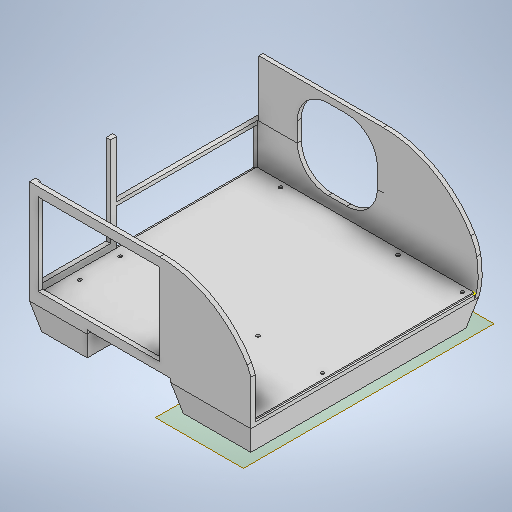
# Autodesk Inventor part: matx-arc-case-r2
Saved by Autodesk Inventor 2025 (Build 290162000, 162)
## iProperties
Created: 2024-07-20
Part Number: matx-arc-case-r2
Material: Generic
Document SubType Name: Modeling
Designer: admin
Density: 1 g/cm^3
Appearance: Default
Author: admin
Autodesk Inventor part; units mm, degrees
ref_plane "YZ Plane" through (0, 0, 0) normal (1, 0, 0) x (0, 1, 0)
ref_plane "XZ Plane" through (0, 0, 0) normal (0, 1, 0) x (-1, 0, 0)
ref_plane "XY Plane" through (0, 0, 0) normal (0, 0, 1) x (1, 0, 0)
sketch "Sketch2" plane through (0, 0, 0) normal (0, 1, 0) x (-1, 0, 0)
  line L0 (0, 0) -> (0, -243.84)
  line L1 (0, -243.84) -> (243.84, -243.84)
  line L2 (243.84, -243.84) -> (243.84, 0)
  line L3 (243.84, 0) -> (0, 0)
  line L4 (243.84, 0) -> (233.68, 0)
  line L5 (233.68, 0) -> (6.35, 0)
  line L6 (233.68, 0) -> (78.74, 0)
  line L7 (233.68, -243.84) -> (210.82, -243.84)
  line L8 (233.68, 0) -> (233.68, -243.84)
  line L9 (243.84, -243.84) -> (243.84, -85.09)
  line L10 (6.35, 0) -> (6.35, -243.84)
  line L11 (78.74, 0) -> (78.74, -243.84)
  line L12 (243.84, -85.09) -> (243.84, -31.85)
  line L13 (78.74, -31.85) -> (78.74, -77.57)
  line L14 (78.74, 0) -> (78.74, -34.29)
  line L15 (78.74, -34.29) -> (78.74, -13.97)
  line L16 (78.74, -34.29) -> (78.74, -80.01)
  circle A0 centre (78.74, -80.01) radius 2
  circle A1 centre (78.74, -34.29) radius 2
  circle A2 centre (78.74, -13.97) radius 2
  circle A3 centre (6.35, -80.01) radius 2
  line L17 (78.74, -34.29) -> (78.74, -237.49)
  circle A4 centre (78.74, -237.49) radius 2
  circle A5 centre (6.35, -237.49) radius 2
  circle A6 centre (210.82, -237.49) radius 2
  circle A7 centre (233.68, -34.29) radius 2
  circle A8 centre (233.68, -80.01) radius 2
  dimension "d79" = 243.84
  dimension "d80" = 243.84
  dimension "d81" = 10.16
  dimension "d82" = 227.33
  dimension "d83" = 154.94
  dimension "d84" = 22.86
  dimension "d85" = 158.75
  dimension "d92" = 34.29
  dimension "d93" = 20.32
  dimension "d94" = 45.72
  dimension "d95" = 203.2
  constraints: 36 end point, 17 point on line, 9 centre point, 4 coincident, 4 perpendicular, 2 vertical, 1 parallel
  measures "d79" distance of L0.start L0.end
  measures "d80" distance of L0.end L1.end
  measures "d81" distance of L2.end L4.end
  measures "d82" distance of L4.end L5.end
  measures "d83" distance of L4.end L6.end
  measures "d84" distance of L7.start L7.end
  measures "d85" distance of L1.end L9.end
  measures "d92" distance of L6.end L14.end
  measures "d93" distance of L14.end L15.end
  measures "d94" distance of L14.end L16.end
  measures "d95" distance of L17.start L17.end
extrude "Extrusion1" add sketch "Sketch2" along normal blind 1.5 contours L3 L10 A3 A5 L1 L0 | L3 L11 A2 A1 A0 A4 L1 L10 A5 A3 | L3 L8 A7 A8 L1 L11 A4 A0 A1 A2 | L3 L2 L1 L8 A8 A7
sketch "Sketch4" plane through (-243.84, 0, -243.84) normal (-1, 0, 0) x (0, 0, 1)
  line L0 (0.0105, -0.4083) -> (0.0105, -1.9083)
  line L1 (243.84, 0) -> (0, 0) projected
  line L2 (0.0105, -1.9083) -> (-1.25, -1.9083)
  line L3 (-1.25, -1.9083) -> (-1.25, 42.5417)
  line L4 (-1.25, -1.9083) -> (43.2, -1.9083) construction
  line L5 (-1.25, 42.5417) -> (157.5, 42.5417)
  line L6 (157.5, 42.5417) -> (157.5, -1.9083)
  line L7 (-1.25, -1.9083) -> (-1.25, -6.0083)
  line L8 (-1.25, -6.0083) -> (157.5, -6.0083)
  line L9 (-1.25, -6.0083) -> (-5.35, -6.0083)
  line L10 (-5.35, -6.0083) -> (-5.35, 42.5417)
  line L11 (-5.35, 42.5417) -> (-5.35, 46.6417)
  line L12 (-5.35, 46.6417) -> (157.5, 46.6417)
  line L13 (157.5, 46.6417) -> (161.6, 46.6417)
  line L14 (161.6, 46.6417) -> (161.6, -1.9083)
  line L15 (161.6, -6.0083) -> (157.5, -6.0083)
  line L16 (161.6, -6.0083) -> (161.6, -1.9083)
  line L17 (0.0105, -1.9083) -> (157.5, -1.9083)
  line L18 (161.6, -6.0083) -> (243.84, -6.0083)
  line L19 (161.6, -6.0083) -> (161.6, 9.1917)
  line L20 (161.6, 9.1917) -> (243.84, 9.1917)
  line L21 (243.84, 9.1917) -> (243.84, -6.0083)
  line L22 (157.5, 42.5417) -> (164.5, 42.5417)
  line L23 (164.5, 42.5417) -> (164.5, 9.1917)
  line L24 (164.5, 42.5417) -> (164.5, 46.6417)
  line L25 (164.5, 46.6417) -> (161.6, 46.6417)
  line L26 (164.5, 9.1917) -> (164.5, 110.1917)
  line L27 (164.5, 110.1917) -> (243.84, 110.1917)
  line L28 (243.84, 110.1917) -> (243.84, 9.1917)
  line L29 (157.5, 46.6417) -> (157.5, 110.1917)
  line L30 (250.84, 110.1917) -> (250.84, -6.0083)
  line L31 (250.84, -6.0083) -> (243.84, -6.0083)
  line L32 (243.84, 110.1917) -> (250.84, 110.1917)
  line L33 (157.5, 110.1917) -> (164.5, 110.1917)
  dimension "d98" = 1.5
  dimension "d103" = 44.45
  dimension "d104" = 90
  dimension "d105" = 158.75
  dimension "d106" = 4.1
  dimension "d107" = 4.1
  dimension "d108" = 4.1
  dimension "d109" = 4.1
  dimension "d110" = 15.2
  dimension "d111" = 7
  dimension "d112" = 101
  constraints: 66 end point, 14 perpendicular, 13 point on line, 3 horizontal, 3 vertical, 2 collinear, 2 parallel
  measures "d98" distance of L0.start L0.end
  measures "d103" distance of L2.end L3.end
  measures "d104" angle of L4 L3
  measures "d105" distance of L3.end L5.end
  measures "d106" distance of L2.end L7.end
  measures "d107" distance of L7.end L9.end
  measures "d108" distance of L10.end L11.end
  measures "d109" distance of L12.end L13.end
  measures "d110" distance of L15.start L19.end
  measures "d111" distance of L5.end L22.end
  measures "d112" distance of L23.end L26.end
extrude "Extrusion2" add sketch "Sketch4" along normal blind 5 contours L21 L18 L16 L14 L1 | L1 L14 L20 L21 | L21 L28 L32 L30 L31 | L14 L16 L15 L8 L7 L2 L17 L6 L1 | L1 L6 L22 L14 | L14 L22 L23 L20 | L5 L3 L7 L9 L10 L11 L12 L13 L14 L22 | L14 L25 L24 L22 | L26 L25 L13 L29 L33
sketch "Sketch5" plane through (-243.84, 0, -243.84) normal (1, 0, 0) x (0, 0, -1)
  line L0 (5.35, -6.0083) -> (-250.84, -6.0083) projected
  line L1 (-250.84, -6.0083) -> (5.35, -6.0083)
  line L2 (5.35, -6.0083) -> (5.35, -1.9083)
  line L3 (5.35, -1.9083) -> (-250.84, -1.9083)
  line L4 (-157.5, -1.9083) -> (1.25, -1.9083) projected
  line L5 (-250.84, -1.9083) -> (-250.84, -6.0083)
  point P0 (-243.84, 0)
  constraints: 8 end point, 2 collinear, 2 perpendicular
extrude "Extrusion3" add sketch "Sketch5" along normal blind 60
sketch "Sketch6" plane through (-248.84, -1.9083, -86.34) normal (0, 1, 0) x (1, 0, 0)
  circle A0 centre (15.16, -52.05) radius 2 projected
  circle A1 centre (15.16, -52.05) radius 2
  circle A2 centre (15.16, -6.33) radius 2 projected
  circle A3 centre (15.16, -6.33) radius 2
  circle A4 centre (37.9882, 151.128) radius 2.0223
  point P0 (248.84, -86.34)
  constraints: 3 centre point, 2 coincident
extrude "Extrusion4" cut sketch "Sketch6" against normal blind 28.25
ref_plane "Work Plane1" through (-248.84, -36.0083, -249.19) normal (0, -1, 0) x (1, 0, 0)
sketch "Sketch7" plane through (-248.84, -36.0083, -249.19) normal (0, -1, 0) x (1, 0, 0)
  line L0 (65, 256.19) -> (65, 0) projected
  line L1 (65, 256.19) -> (65, 249.19)
  line L2 (7, 249.19) -> (7, 7)
  line L3 (7, 7) -> (58, 7)
  line L4 (58, 7) -> (58, 249.19)
  line L5 (58, 249.19) -> (7, 249.19)
  line L6 (5, 249.19) -> (248.84, 249.19) projected
  dimension "d122" = 7
  constraints: 10 end point, 2 perpendicular, 1 collinear, 1 point on line
  measures "d122" distance of L1.end L4.end
loft "Loft1" add profiles "Sketch7" section 2 edges at (-216.34, -6.0083, 7) (-248.84, -6.0083, -121.095) (-216.34, -6.0083, -249.19) (-183.84, -6.0083, -121.095)
ref_plane "Work Plane2" through (0.16, 0, -243.84) normal (1, 0, 0) x (0, 0, -1)
sketch "Sketch8" plane through (0.16, 0, -243.84) normal (1, 0, 0) x (0, 0, -1)
  line L0 (5.35, -1.9083) -> (-250.84, -1.9083) projected
  line L1 (-250.84, -1.9083) -> (5.35, -1.9083)
  line L2 (5.35, -6.0083) -> (-250.84, -6.0083) projected
  line L3 (5.35, -1.9083) -> (5.35, -6.0083)
  line L4 (5.35, -6.0083) -> (-250.84, -6.0083)
  line L5 (-250.84, -6.0083) -> (-250.84, -1.9083)
  point P0 (-243.84, 0)
  constraints: 8 end point, 3 perpendicular, 1 horizontal
extrude "Extrusion5" add sketch "Sketch8" against normal blind 90
ref_plane "Work Plane3" through (0.16, -36.0083, -249.19) normal (0, -1, 0) x (1, 0, 0)
sketch "Sketch9" plane through (0.16, -36.0083, -249.19) normal (0, -1, 0) x (1, 0, 0)
  line L0 (0, 256.19) -> (-90, 256.19) projected
  line L1 (-90, 256.19) -> (-90, 0) projected
  line L2 (-83, 249.19) -> (-7, 249.19)
  line L3 (-7, 249.19) -> (-7, 7)
  line L4 (0, 0) -> (-90, 0) projected
  line L5 (-83, 7) -> (-7, 7)
  line L6 (-83, 7) -> (-83, 249.19)
  constraints: 8 end point, 1 perpendicular
loft "Loft2" add profiles "Sketch9" section 2 edges at (0.16, -6.0083, -121.095) (-44.84, -6.0083, 7) (-89.84, -6.0083, -121.095) (-44.84, -6.0083, -249.19)
sketch "Sketch10" plane through (-248.84, -1.9083, -86.34) normal (0, 1, 0) x (1, 0, 0)
  line L0 (5, 158.75) -> (5, 162.85) projected
  line L1 (242, 155.85) -> (249, 162.85) projected
  line L2 (5, 162.85) -> (249, 162.85)
  line L3 (249, 162.85) -> (249, 158.35)
  line L4 (249, 158.35) -> (5, 158.35)
  line L5 (5, 158.35) -> (5, 162.85)
  point P0 (248.84, -86.34)
  point P1 (244.5, 158.35)
  dimension "d142" = 4.5
  constraints: 8 end point, 3 perpendicular, 1 horizontal
  measures "d142" distance of L1.end L3.end
extrude "Extrusion6" add sketch "Sketch10" along normal blind 48.54
sketch "Sketch11" plane through (-183.84, -1.9083, -244.69) normal (0, 0, 1) x (1, 0, 0)
  point P0 (183.84, 1.9083)
sketch "Sketch12" plane through (-183.84, -6.0083, -249.19) normal (0, 0, -1) x (-1, 0, 0)
  line L0 (65, 116.2) -> (65, 52.65) projected
  line L1 (65, 52.65) -> (65, 116.2)
  line L2 (65, 116.2) -> (58.6377, 116.2)
  line L3 (58.6377, 116.2) -> (58.6377, 52.65)
  line L4 (58.6377, 52.65) -> (-81.3623, 52.64)
  line L5 (60, 52.64) -> (-184, 52.64) projected
  line L6 (58.6377, 116.2) -> (-81.3623, 116.2)
  line L7 (-81.3623, 116.2) -> (-81.3623, 52.64)
  line L8 (-179.5, 52.64) -> (-184, 52.64) projected
  arc A0 (-81.3623, 116.2) -> (-184, 52.64) centre (-81.3623, 1.5495) ccw
  line L9 (-184, 4.1) -> (-184, 52.64) projected
  arc A1 (-184, 52.64) -> (-184, -0.3678) centre (-99.2421, 26.1361) ccw
  line L10 (-184, -0.3678) -> (-184, 52.64)
  line L11 (-184, 4.1) -> (-184, 0) projected
  point P0 (-183.84, 6.0083)
  dimension "d145" = 140
  constraints: 14 end point, 4 point on circle, 3 perpendicular, 2 centre point, 1 collinear, 1 horizontal, 1 point on line, 1 tangent, 1 vertical
  measures "d145" distance of L3.end L4.end
extrude "Extrusion7" add sketch "Sketch12" against normal blind 4.5
fillet "Fillet1" radius 53.25 1 edges at (0.16, 46.6317, -246.94)
sketch "Sketch13" plane through (-183.84, -6.0083, -249.19) normal (0, 0, -1) x (-1, 0, 0)
  line L0 (-74.6961, 108.9977) -> (-74.6961, 18.9977)
  line L1 (-74.6961, 18.9977) -> (15.3039, 18.9977)
  line L2 (15.3039, 18.9977) -> (15.3039, 108.9977)
  line L3 (58.6377, 116.2) -> (-81.3623, 116.2) projected
  line L4 (15.3039, 108.9977) -> (-74.6961, 108.9977)
  point P0 (-183.84, 6.0083)
  dimension "d149" = 90
  dimension "d150" = 90
  constraints: 8 end point, 3 perpendicular, 1 vertical
  measures "d149" distance of L0.start L0.end
  measures "d150" distance of L0.end L1.end
extrude "Extrusion8" cut sketch "Sketch13" against normal blind 24.5
fillet "Fillet2" radius 34.5 4 edges at (-199.1439, 12.9894, -246.94) (-199.1439, 102.9894, -246.94) (-109.1439, 102.9894, -246.94) (-109.1439, 12.9894, -246.94)
sketch "Sketch14" plane through (-89.84, -1.9083, 7) normal (0, 1, 0) x (1, 0, 0)
  line L0 (-154, 0) -> (-154, 93.34) projected
  line L1 (90, 0) -> (0, 0) projected
  line L2 (-154, 0) -> (90, 0)
  line L3 (90, 0) -> (90, 5)
  line L4 (90, 5) -> (-154, 5)
  line L5 (-154, 5) -> (-154, 0)
  point P0 (89.84, 7)
  dimension "d154" = 5
  constraints: 8 end point, 3 perpendicular, 1 horizontal
  measures "d154" distance of L1.start L3.end
extrude "Extrusion9" add sketch "Sketch14" along normal blind 112.1
sketch "Sketch15" plane through (-89.84, -1.9083, 2) normal (0, 0, -1) x (-1, 0, 0)
  line L0 (152.6377, 112.1) -> (12.6377, 112.1) projected
  arc A0 (12.6377, 112.1) -> (-85.9195, 56.0261) centre (12.6377, -2.5505) ccw projected
  arc A1 (12.6377, 112.1) -> (-85.9195, 56.0261) centre (12.6377, -2.5505) ccw
  arc A2 (-92.4159, 38.9798) -> (-90, -4.4678) centre (-5.2421, 22.0361) ccw projected
  arc A3 (-85.9195, 56.0261) -> (-90, -4.4678) centre (-13.3257, 20.7448) ccw
  line L1 (-90, 112.1) -> (159, 112.1) projected
  line L2 (-90, -4.4678) -> (-90, 112.1)
  line L3 (-90, 112.1) -> (12.6377, 112.1)
  point P0 (-89.84, 1.9083)
  point P1 (-90, 45.9575)
  constraints: 4 end point, 4 point on circle, 2 centre point, 1 collinear, 1 vertical
extrude "Extrusion10" cut sketch "Sketch15" against normal blind 16.4 contours A0 A3 L2 L1
sketch "Sketch16" plane through (-89.84, -1.9083, 2) normal (0, 0, -1) x (-1, 0, 0)
  line L0 (12.6377, 112.1) -> (159, 112.1) projected
  line L1 (159, 112.1) -> (159, 102.1)
  line L2 (159, -4.1) -> (159, 112.1) projected
  line L3 (12.6377, 102.1) -> (12.6377, -0.0079)
  line L4 (12.6377, -0.0079) -> (12.6377, 9.9921)
  line L5 (12.6377, 9.9921) -> (149, 9.9921)
  line L6 (149, 9.9921) -> (149, 102.1)
  line L7 (149, 102.1) -> (12.6377, 102.1)
  arc A0 (-85.9195, 56.0261) -> (-90, 45.9575) centre (-13.3257, 20.7448) ccw projected
  point P0 (-89.84, 1.9083)
  dimension "d152" = 0
  dimension "d160" = 10
  constraints: 12 end point, 2 point on line, 1 horizontal, 1 perpendicular
  measures "d160" distance of L3.end L4.end
extrude "Extrusion11" cut sketch "Sketch16" against normal blind 16.4
body "Solid1"
